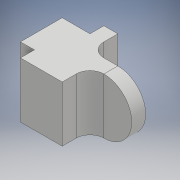
# Autodesk Inventor part: 21
Saved by Autodesk Inventor 2017 (Build 210142000, 142)
## iProperties
Part Number: 21
Material: 一般
Document SubType Name: Modeling
Designer: Brian
Density: 1 g/cm^3
Appearance: 預設
Author: Brian
Autodesk Inventor part; units mm, degrees
ref_plane "YZ Plane" through (0, 0, 0) normal (1, 0, 0) x (0, 1, 0)
ref_plane "XZ Plane" through (0, 0, 0) normal (0, 1, 0) x (-1, 0, 0)
ref_plane "XY Plane" through (0, 0, 0) normal (0, 0, 1) x (1, 0, 0)
sketch "草圖1" plane through (0, 0, 0) normal (0, 0, 1) x (1, 0, 0)
  line L0 (0, 0) -> (30, 0)
  line L1 (30, 0) -> (30, 10)
  line L2 (30, 10) -> (0, 10)
  line L3 (0, 10) -> (0, 0)
  line L4 (30, 10) -> (-10, 10)
  line L5 (-10, 10) -> (-10, 20)
  line L6 (-10, 20) -> (30, 20)
  line L7 (30, 20) -> (30, 10)
  line L8 (-10, 20) -> (60, 20)
  line L9 (60, 20) -> (60, 30)
  line L10 (60, 30) -> (-10, 30)
  line L11 (-10, 30) -> (-10, 20)
  line L12 (-10, 30) -> (20, 30)
  line L13 (20, 30) -> (20, 40)
  line L14 (20, 40) -> (-10, 40)
  line L15 (-10, 40) -> (-10, 30)
  line L16 (20, 40) -> (10, 40)
  line L17 (10, 40) -> (10, 50)
  line L18 (10, 50) -> (20, 50)
  line L19 (20, 50) -> (20, 40)
  dimension "d0" = 10
  dimension "d1" = 10
  dimension "d2" = 10
  dimension "d3" = 10
  dimension "d4" = 10
  dimension "d5" = 30
  dimension "d6" = 10
  dimension "d7" = 70
  dimension "d8" = 30
  dimension "d9" = 10
  constraints: 40 end point, 10 parallel, 5 horizontal, 5 perpendicular
  measures "d0" distance of L16.end L17.end
  measures "d1" distance of L14.end L10.end
  measures "d2" distance of L10.end L5.end
  measures "d3" distance of L4.end L5.end
  measures "d4" distance of L2.end L0.start
  measures "d5" distance of L0.start L0.end
  measures "d6" distance between parallel lines of L3 L5
  measures "d7" distance of L5.end L8.end
  measures "d8" distance of L13.end L14.end
  measures "d9" distance of L17.end L18.end
extrude "擠出1" add sketch "草圖1" along normal blind 40
fillet "圓角1" radius 20 2 edges at (60, 25, 40) (60, 25, 0)
fillet "圓角2" radius 10 2 edges at (20, 30, 20) (30, 20, 20)
